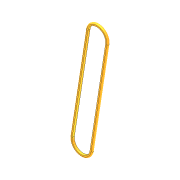
# Autodesk Inventor part: Belt_VerticalConveyor_Outer
Saved by Autodesk Inventor 2012 (Build 160160000, 160)
## iProperties
Created: 2012-01-21
Part Number: Belt_VerticalConveyor_Outer
Material: Default
Document SubType Name: Modeling
Designer: JesseK
Density: 1 g/cm^3
Author: JesseK
Autodesk Inventor part; units mm, degrees
ref_plane "YZ Plane" through (0, 0, 0) normal (1, 0, 0) x (0, 1, 0)
ref_plane "XZ Plane" through (0, 0, 0) normal (0, 1, 0) x (-1, 0, 0)
ref_plane "XY Plane" through (0, 0, 0) normal (0, 0, 1) x (1, 0, 0)
sketch "Sketch1" plane through (0, 0, 0) normal (0, 0, 1) x (1, 0, 0)
  arc A0 (18.8233, -2.9299) -> (-18.8233, 2.9299) centre (0, 0) ccw
  arc A1 (-52.0289, -210.4013) -> (-14.3822, -216.2611) centre (-33.2055, -213.3312) ccw
  line L0 (0, 0) -> (-33.2055, -213.3312) construction
  line L1 (18.8233, -2.9299) -> (-14.3822, -216.2611)
  line L2 (-18.8233, 2.9299) -> (-52.0289, -210.4013)
  line L3 (-33.2055, -213.3312) -> (-14.3822, -216.2611) construction
  line L4 (0, 0) -> (18.8233, -2.9299) construction
  arc A2 (23.5292, -3.6624) -> (-23.5292, 3.6624) centre (0, 0) ccw
  arc A3 (-56.7347, -209.6688) -> (-9.6763, -216.9936) centre (-33.2055, -213.3312) ccw
  line L5 (-23.5292, 3.6624) -> (-56.7347, -209.6688)
  line L6 (-9.6763, -216.9936) -> (23.5292, -3.6624)
  dimension "d0" = 215.9
  dimension "d1" = 4.7625
  dimension "d2" = 19.05
  constraints: 14 end point, 8 point on circle, 8 tangent, 4 centre point, 3 coincident, 3 parallel, 1 perpendicular
  measures "d0" distance between parallel lines of L3 L4
  measures "d1" radial gap between concentric circles of A2 A0
  measures "d2" radius of A0
extrude "Extrusion1" add sketch "Sketch1" along normal blind 4.7625
fillet "Fillet1" radius 2.3813 8 edges at (-36.8679, -236.8604, 4.7625) (-40.1319, -103.0032, 4.7625) (3.6624, 23.5292, 4.7625) (6.9264, -110.328, 4.7625) (3.6624, 23.5292, 0) (-40.1319, -103.0032, 0) (-36.8679, -236.8604, 0) (6.9264, -110.328, 0)
body "Solid1"
